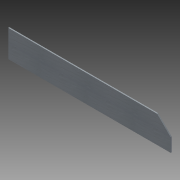
# Autodesk Inventor part: Side_Panel
Saved by Autodesk Inventor 2011 SP1 (Build 150282100, 282)
## iProperties
Created: 2011-05-30
Part Number: Side_Panel
Document SubType Name: Modeling
Designer: Andrew G. Meyer
Mass: 108.308 g
Surface Area: 715.419 cm^2
Volume: 108.308 cm^3
Density: 1 g/cm^3
Author: Andrew G. Meyer
Autodesk Inventor part; units mm, degrees
ref_plane "YZ Plane" through (0, 0, 0) normal (1, 0, 0) x (0, 1, 0)
ref_plane "XZ Plane" through (0, 0, 0) normal (0, 1, 0) x (-1, 0, 0)
ref_plane "XY Plane" through (0, 0, 0) normal (0, 0, 1) x (1, 0, 0)
sketch "Sketch1" plane through (0, 0, 0) normal (0, 0, 1) x (1, 0, 0)
  line L0 (-228.6, 38.1) -> (190.5, 38.1)
  line L1 (228.6, 0) -> (228.6, -38.1)
  line L2 (228.6, -38.1) -> (-228.6, -38.1)
  line L3 (-228.6, -38.1) -> (-228.6, 38.1)
  line L4 (190.5, 38.1) -> (228.6, 0)
  point P0 (0, 0)
  dimension "d1" = 76.2
  dimension "d2" = 38.1
  dimension "d3" = 228.6
  dimension "d6" = 38.1
  dimension "d7" = 45
  dimension "d8" = 457.2
  constraints: 10 end point, 2 parallel, 1 horizontal, 1 perpendicular
  measures "d1" distance of L2.end L0.start
  measures "d2" distance from line of L0 point (0, 0)
  measures "d3" distance from line of L3 point (0, 0)
  measures "d6" distance of L1.end L1.start
  measures "d7" angle of L1 L4
  measures "d8" distance of L1.end L2.end
extrude "Extrusion1" add sketch "Sketch1" against normal blind 3.175
body "Solid1"
